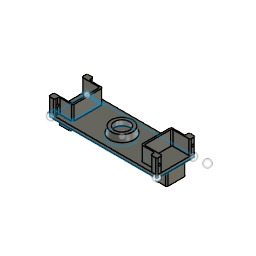
Servo_holder (Autodesk Fusion 360 archive; units mm, degrees)
design "Servo_holder" references "Towerpro Micro Servo 9g"
part number: 2026-08-20-22-19-28-924
Autodesk Fusion 360 part; units mm, degrees
sketch "Sketch1" plane through (0, 0, 0) normal (0, 0, 1) x (1, 0, 0)
  circle A0 centre (-45.0484, 12.8566) radius 10
  line L0 (-90.0484, 24.9) -> (-90.0484, 27.8566)
  line L1 (-0.0484, 24.9) -> (-0.0484, 27.8566)
  arc A1 (-89.0484, 28.8566) -> (-90.0484, 27.8566) centre (-89.0484, 27.8566) ccw
  line L2 (-90.0484, 24.9) -> (-90.0484, -2.1434)
  arc A2 (-90.0484, -2.1434) -> (-89.0484, -3.1434) centre (-89.0484, -2.1434) ccw
  arc A3 (-0.0484, 27.8566) -> (-1.0484, 28.8566) centre (-1.0484, 27.8566) ccw
  line L3 (-89.0484, 28.8566) -> (-1.0484, 28.8566)
  line L4 (-0.0484, 24.9) -> (-0.0484, -2.13)
  arc A4 (-1.0646, -3.1299) -> (-0.0484, -2.13) centre (-1.0484, -2.13) ccw
  line L5 (-1.0646, -3.1299) -> (-89.0484, -3.1434)
  point P0 (-90.0484, 28.8566)
  point P1 (9.9516, 28.8566)
  dimension "d1" = 100
  dimension "d6" = 20
  dimension "d45" = 1
  dimension "d46" = 1
  dimension "d47" = 1
  constraint tangent L0 A1
  constraint tangent L2 A2
  constraint tangent L1 A3
  constraint equal A2 A3
  constraint tangent A3 L3
  constraint tangent L4 A4
  measures "d1" distance of P0 P1
  measures "d6" diameter of A0
  measures "d45" radius of A1
  measures "d46" radius of A2
  measures "d47" radius of A4
extrude "Extrude2" add sketch "Sketch1" along normal blind 2.5 makes body 1
ref_plane "WorkPlane1" through (-45.0484, 12.8566, 2.5) normal (0, 0, 1) x (1, 0, 0)
sketch "Sketch2" plane through (0, 0, 2.5) normal (0, 0, 1) x (1, 0, 0)
sketch "Sketch4" plane through (0, 0, 2.5) normal (0, 0, 1) x (1, 0, 0)
  line L0 (-90.0484, 28.8566) -> (-90.0484, 24.3566)
  line L1 (-90.0484, 24.3566) -> (-74.9484, 24.3566)
  line L2 (-74.9484, 24.3566) -> (-74.9484, 1.3566)
  line L3 (-74.9484, 1.3566) -> (-90.0484, 1.3566)
  line L4 (-90.0484, 1.3566) -> (-90.0484, -3.1434)
  line L5 (-90.0484, -3.1434) -> (-84.9484, -3.1434)
  line L6 (-84.9484, -3.1434) -> (-84.9484, 0.3566)
  line L7 (-84.9484, 0.3566) -> (-73.4484, 0.3566)
  line L8 (-73.4484, 0.3566) -> (-73.4484, 25.3566)
  line L9 (-73.4484, 25.3566) -> (-84.7772, 25.3566)
  line L10 (-84.7772, 25.3566) -> (-84.7772, 28.8566)
  line L11 (-84.7772, 28.8566) -> (-90.0484, 28.8566)
  constraint vertical L0
  constraint perpendicular L0 L1
  constraint perpendicular L1 L2
  constraint perpendicular L2 L3
  constraint perpendicular L3 L4
  constraint perpendicular L4 L5
  constraint perpendicular L5 L6
  constraint perpendicular L6 L7
  constraint perpendicular L7 L8
  constraint perpendicular L0 L9
  constraint perpendicular L9 L10
  constraint perpendicular L0 L11
extrude "Extrude4" add sketch "Sketch4" along normal blind 12 separate body makes body 2
fillet "Fillet1" radius 1 1 edges at (-74.9484, 24.3566, 8.5) on bodies 2
fillet "Fillet2" radius 1 1 edges at (-74.9484, 1.3566, 8.5) on bodies 2
fillet "Fillet3" radius 1 1 edges at (-90.0484, 24.3566, 8.5) on bodies 2
fillet "Fillet4" radius 1 1 edges at (-90.0484, 1.3566, 8.5) on bodies 2
fillet "Fillet5" radius 1 1 edges at (-90.0484, -3.1434, 8.5) on bodies 2
fillet "Fillet6" radius 1 1 edges at (-90.0484, 28.8566, 8.5) on bodies 2
fillet "Fillet7" radius 1 1 edges at (-84.9484, -3.1434, 8.5) on bodies 2
fillet "Fillet8" radius 1 1 edges at (-84.9484, 0.3566, 8.5) on bodies 2
fillet "Fillet9" radius 1 1 edges at (-73.4484, 0.3566, 8.5) on bodies 2
fillet "Fillet10" radius 1 1 edges at (-73.4484, 25.3566, 8.5) on bodies 2
fillet "Fillet11" radius 1 1 edges at (-84.7772, 25.3566, 8.5) on bodies 2
fillet "Fillet12" radius 1 1 edges at (-84.7772, 28.8566, 8.5) on bodies 2
fillet "Fillet13" [no effect]
copy_body "CopyPasteBodies1" bodies 2 makes body 3
move_body "Move1" bodies 3 to x (-1, 0, 0) y (0, -1, 0) z (0, 0, 1) at (-90.1109, 25.7382, 0)
ref_plane "WorkPlane2" through (-45.0484, 12.8566, 7.5) normal (0, 0, 1) x (1, 0, 0)
sketch "Sketch5" plane through (0, 0, 7.5) normal (0, 0, 1) x (1, 0, 0)
  circle A0 centre (-45.0484, 12.8566) radius 8.75
  point P0 (-45.0484, 12.8566)
  dimension "d50" = 17.5
  constraint coincident P0 A0.centre
  measures "d50" diameter of A0
loft "Loft1" add profiles "Sketch1", "Sketch5" section 1 contours A0 section 2 separate body makes body 4
shell "Shell1" thickness 2.5 removed faces 1 at (-42.8372, 9.896, 7.5) on bodies 4
ref_plane "WorkPlane3" through (-45.0484, 12.8566, 0) normal (0, 0, 1) x (1, 0, 0)
sketch "Sketch6" plane through (0, 0, 0) normal (0, 0, 1) x (1, 0, 0)
  line L0 (-90, 5) -> (-81, 5)
  line L1 (-80, 6) -> (-80, 20)
  line L2 (-81, 21) -> (-90, 21)
  line L3 (-90, 21) -> (-90, 5)
  line L4 (0, 5) -> (-9, 5)
  line L5 (-10, 6) -> (-10, 20)
  line L6 (-9, 21) -> (0, 21)
  line L7 (0, 21) -> (0, 5)
  arc A0 (-10, 6) -> (-9, 5) centre (-9, 6) ccw
  arc A1 (-9, 21) -> (-10, 20) centre (-9, 20) ccw
  arc A2 (-81, 5) -> (-80, 6) centre (-81, 6) ccw
  arc A3 (-80, 20) -> (-81, 21) centre (-81, 20) ccw
  dimension "d56" = 16
  dimension "d57" = 16
  dimension "d58" = 1
  constraint perpendicular L0 L1
  constraint parallel L0 L2
  constraint parallel L1 L3
  constraint horizontal L0
  constraint perpendicular L4 L5
  constraint parallel L4 L6
  constraint parallel L5 L7
  constraint perpendicular L1 L4
  constraint tangent L4 A0
  constraint tangent L5 A0
  constraint tangent L5 A1
  constraint tangent L6 A1
  constraint equal A0 A1
  constraint tangent L0 A2
  constraint tangent L1 A2
  constraint equal A0 A2
  constraint tangent L1 A3
  constraint tangent L2 A3
  constraint equal A0 A3
  measures "d56" distance of L0.start L2.end
  measures "d57" distance of L4.start L6.end
  measures "d58" radius of A0
extrude "Extrude5" add sketch "Sketch6" against normal blind 10 separate body makes body 5 at (-90, 15.6667, -3.3333) makes body 6 at (0, 15.6667, -3.3333)
fillet "Fillet14" radius 1 1 edges at (-90, 21, -5) on bodies 5
fillet "Fillet15" radius 1 1 edges at (-90, 5, -5) on bodies 5
fillet "Fillet16" radius 1 1 edges at (0, 21, -5) on bodies 6
fillet "Fillet17" radius 1 1 edges at (0, 5, -5) on bodies 6
ref_plane "WorkPlane4" through (-90.0484, 12.8566, 8.5) normal (-1, 0, 0) x (0, -1, 0)
sketch "Sketch7" plane through (-90.0484, 0, 0) normal (-1, 0, 0) x (0, -1, 0)
  circle A0 centre (-26.6136, 8.9902) radius 1.0629
  circle A1 centre (0.9864, 8.9902) radius 1.0629
extrude "Extrude6" cut sketch "Sketch7" against normal blind 92 bodies 2 3
extrude "Extrude3" [suppressed]
extrude "Extrude1" [suppressed]
